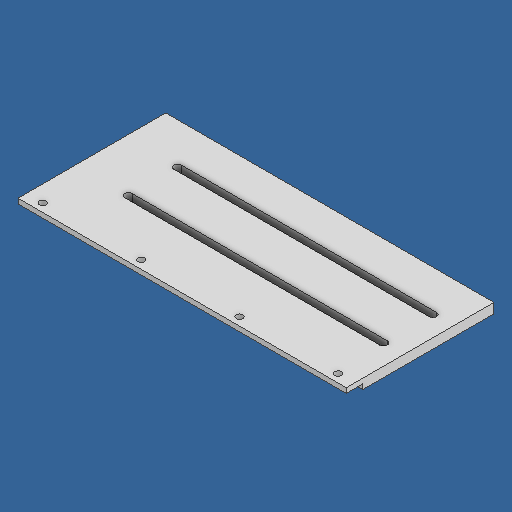
# Autodesk Inventor part: MesaDePruebas
Saved by Autodesk Inventor 2025 (Build 290162000, 162)
## iProperties
Created: 2025-09-23
Part Number: MesaDePruebas
Material: Genérico
Document SubType Name: Modeling
Designer: HP
Density: 1 g/cm^3
Appearance: Valor por defecto
Author: HP
Autodesk Inventor part; units mm, degrees
ref_plane "YZ Plane" through (0, 0, 0) normal (1, 0, 0) x (0, 1, 0)
ref_plane "XZ Plane" through (0, 0, 0) normal (0, 1, 0) x (-1, 0, 0)
ref_plane "XY Plane" through (0, 0, 0) normal (0, 0, 1) x (1, 0, 0)
sketch "Boceto1" plane through (0, 0, 0) normal (0, 1, 0) x (-1, 0, 0)
  line L0 (-100, 40) -> (100, 40)
  line L1 (100, 40) -> (100, -40)
  line L2 (100, -40) -> (-100, -40)
  line L3 (-100, -40) -> (-100, 40)
  line L4 (-100, 40) -> (100, -40) construction
  line L5 (100, 40) -> (-100, -40) construction
  point P0 (0, 0)
  dimension "d0" = 200
  dimension "d1" = 80
  constraints: 12 end point, 2 midpoint, 2 parallel, 1 horizontal, 1 perpendicular
  measures "d0" distance of L1.end L2.end
  measures "d1" distance of L0.end L1.end
extrude "Extrusión1" add sketch "Boceto1" along normal blind 6
sketch "Boceto2" plane through (0, 6, 0) normal (0, 1, 0) x (1, 0, 0)
  line L0 (-67.75, -17.25) -> (87.75, -17.25)
  line L1 (90, -15) -> (90, -15)
  line L2 (87.75, -12.75) -> (-67.75, -12.75)
  line L3 (-70, -15) -> (-70, -15)
  line L4 (0, 0) -> (-99.8063, 0) construction
  line L5 (100, -40) -> (100, 40) construction
  line L6 (100, 40) -> (-100, 40) construction
  line L7 (-100, 40) -> (-100, -40) construction
  line L8 (-100, -40) -> (100, -40) construction
  line L9 (100, -40) -> (100, 40) construction
  arc A0 (-70, -15) -> (-67.75, -17.25) centre (-67.75, -15) ccw
  arc A1 (-67.75, -12.75) -> (-70, -15) centre (-67.75, -15) ccw
  arc A2 (87.75, -17.25) -> (90, -15) centre (87.75, -15) ccw
  arc A3 (90, -15) -> (87.75, -12.75) centre (87.75, -15) ccw
  line L10 (-67.75, 17.25) -> (87.75, 17.25)
  line L11 (87.75, 12.75) -> (-67.75, 12.75)
  arc A4 (-67.75, 17.25) -> (-70, 15) centre (-67.75, 15) ccw
  arc A5 (-70, 15) -> (-67.75, 12.75) centre (-67.75, 15) ccw
  arc A6 (90, 15) -> (87.75, 17.25) centre (87.75, 15) ccw
  arc A7 (87.75, 12.75) -> (90, 15) centre (87.75, 15) ccw
  dimension "d4" = 12.75
  dimension "d5" = 4.5
  dimension "d6" = 10
  dimension "d7" = 30
  dimension "d8" = 2.25
  dimension "d9" = 2.25
  dimension "d10" = 2.25
  constraints: 16 point on circle, 14 end point, 12 symmetric about line, 8 centre point, 8 tangent, 2 horizontal, 2 parallel, 1 concentric, 1 midpoint, 1 perpendicular, 4 other
  measures "d4" distance from line of L2 L4.start
  measures "d5" distance between parallel lines of L0 L2
  measures "d6" distance from line of L5 point (90, -15)
  measures "d7" distance between parallel lines of L7 L3
  measures "d8" radius of A0
  measures "d9" radius of A1
  measures "d10" radius of A2
extrude "Extrusión2" cut sketch "Boceto2" against normal blind 6
sketch "Boceto3" plane through (0, 6, 0) normal (0, 1, 0) x (1, 0, 0)
  line L0 (-67.75, -12.75) -> (87.75, -12.75) projected
  arc A0 (87.75, -17.25) -> (87.75, -12.75) centre (87.75, -15) ccw projected
  line L1 (87.75, -17.25) -> (-67.75, -17.25) projected
  arc A1 (-67.75, -12.75) -> (-67.75, -17.25) centre (-67.75, -15) ccw projected
  arc A2 (-67.75, 17.25) -> (-67.75, 12.75) centre (-67.75, 15) ccw projected
  line L2 (-67.75, 17.25) -> (87.75, 17.25) projected
  arc A3 (87.75, 12.75) -> (87.75, 17.25) centre (87.75, 15) ccw projected
  line L3 (87.75, 12.75) -> (-67.75, 12.75) projected
  line L4 (100, 40) -> (-100, 40) projected
  line L5 (-100, 40) -> (-100, -40) projected
  line L6 (-100, -40) -> (100, -40) projected
  line L7 (100, -40) -> (100, 40) projected
  line L8 (-100, -40) -> (100, -40)
  line L9 (100, -40) -> (100, -50)
  line L10 (100, -50) -> (-100, -50)
  line L11 (-100, -50) -> (-100, -40)
  point P0 (0, 0)
  dimension "d13" = 10
  constraints: 8 end point, 2 parallel, 1 horizontal, 1 perpendicular
  measures "d13" distance of L8.end L9.end
extrude "Extrusión3" add sketch "Boceto3" against normal blind 3 contours L9 L10 L11 L6
sketch "Boceto4" plane through (0, 6, 0) normal (0, 1, 0) x (1, 0, 0)
  line L0 (-100, -50) -> (100, -50) projected
  line L1 (-100, -45) -> (100, -45) construction
  circle A0 centre (-90, -45) radius 2
  line L2 (-100, 40) -> (-100, -50) projected
  circle A1 centre (-30, -45) radius 2
  circle A2 centre (30, -45) radius 2
  circle A3 centre (90, -45) radius 2
  point P0 (0, 0)
  dimension "d16" = 5
  dimension "d17" = 4
  dimension "d18" = 10
  dimension "d21" = 60
  constraints: 4 centre point, 2 end point, 1 horizontal, 1 parallel, 1 point on line, 6 other
  measures "d16" distance between parallel lines of L0 L1
  measures "d17" diameter of A0
  measures "d18" distance from line of L2 A0.centre
  measures "d21" distance of A0.centre A1.centre
extrude "Extrusión4" cut sketch "Boceto4" against normal blind 3
